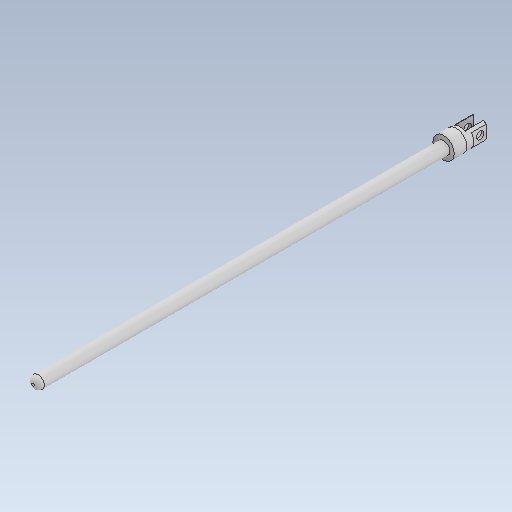
# Autodesk Inventor part: Peça32
Saved by Autodesk Inventor 2021 (Build 250183000, 183)
## iProperties
Category: 41
Created: 2021-07-21
Part Number: Peça32
Material: Genérico
Document SubType Name: Modeling
Designer: Giovanni
Density: 1 g/cm^3
Appearance: Padrão
User Status: 1:2
Author: Giovanni
Keywords: 31
Autodesk Inventor part; units mm, degrees
ref_plane "YZ Plane" through (0, 0, 0) normal (1, 0, 0) x (0, 1, 0)
ref_plane "XZ Plane" through (0, 0, 0) normal (0, 1, 0) x (-1, 0, 0)
ref_plane "XY Plane" through (0, 0, 0) normal (0, 0, 1) x (1, 0, 0)
sketch "Esboço1" plane through (0, 0, 0) normal (0, 0, 1) x (1, 0, 0)
  circle A0 centre (0, 0) radius 8.5
  dimension "d0" = 17
  constraints: 1 centre point, 1 coincident
  measures "d0" diameter of A0
extrude "Extrusão1" add sketch "Esboço1" against normal blind 10
sketch "Esboço2" plane through (0, 0, 0) normal (0, 0, 1) x (1, 0, 0)
  circle A0 centre (0, 0) radius 8.5 projected
  circle A1 centre (0, 0) radius 5
  dimension "d3" = 10
  constraints: 1 centre point, 1 coincident
  measures "d3" diameter of A1
extrude "Extrusão2" add sketch "Esboço2" along normal blind 325 contours A1
sketch "Esboço3" plane through (0, 0, -10) normal (0, 0, -1) x (-1, 0, 0)
  circle A0 centre (0, 0) radius 8.5 projected
  circle A1 centre (0, 0) radius 8
  dimension "d6" = 16
  constraints: 1 centre point, 1 coincident
  measures "d6" diameter of A1
extrude "Extrusão3" add sketch "Esboço3" along normal blind 18 contours A1
sketch "Esboço4" plane through (0, 0, -28) normal (0, 0, -1) x (-1, 0, 0)
  circle A0 centre (0, 0) radius 8 projected
  circle A1 centre (0, 0) radius 8 projected
  line L0 (-4, 6.9282) -> (-4, -6.9282)
  line L1 (4, 6.9282) -> (4, -6.9282)
  arc A2 (-4, -6.9282) -> (4, -6.9282) centre (0, 0) ccw
  arc A3 (4, 6.9282) -> (-4, 6.9282) centre (0, 0) ccw
  point P0 (-4, -6.9282)
  dimension "d9" = 4
  dimension "d10" = 4
  constraints: 8 point on circle, 4 end point, 2 centre point, 1 coincident, 1 vertical
  measures "d9" distance from line of A0.centre L0
  measures "d10" distance from line of L1 A0.centre
extrude "Extrusão4" cut sketch "Esboço4" against normal blind 15 contours L1 A0 L0
sketch "Esboço6" plane through (0, 0, -28) normal (0, 0, -1) x (-1, 0, 0)
  line L0 (-4, -6.9282) -> (-4, 6.9282) projected
  arc A0 (-4, 6.9282) -> (-4, -6.9282) centre (0, 0) ccw projected
  circle A1 centre (0, 0) radius 8 projected
  line L1 (-6, 5.2915) -> (-6, -5.2915)
  line L2 (6, 5.2915) -> (6, -5.2915)
  arc A2 (-6, 5.2915) -> (-6, -5.2915) centre (0, 0) ccw
  arc A3 (6, -5.2915) -> (6, 5.2915) centre (0, 0) ccw
  point P0 (6, -5.2915)
  dimension "d15" = 6
  dimension "d16" = 6
  constraints: 7 point on circle, 6 end point, 2 centre point, 2 vertical, 1 coincident
  measures "d15" distance from line of A0.centre L1
  measures "d16" distance from line of L2 A0.centre
extrude "Extrusão5" cut sketch "Esboço6" against normal blind 12 contours A0 L1 | L2 A1
sketch "Esboço7" plane through (0, 0, 0) normal (1, 0, 0) x (0, 1, 0)
  circle A0 centre (0, -23) radius 3
  line L0 (-6.9282, -28) -> (6.9282, -28) projected
  point P0 (0, 0)
  dimension "d19" = 5
  dimension "d20" = 6
  constraints: 1 centre point, 1 vertical alignment
  measures "d19" distance from line of A0.centre L0
  measures "d20" diameter of A0
extrude "Extrusão6" cut sketch "Esboço7" along normal through all both and the other way through all
chamfer "Chanfro1" distance 0.5 angle 45 4 edges at (-5.0665, -6.1911, -28) (-5.0665, 6.1911, -28) (5.0665, -6.1911, -28) (5.0665, 6.1911, -28)
fillet "Arredondamento1" radius 4 1 edges at (-5, 0, 325)
